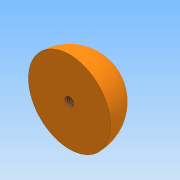
# Autodesk Inventor part: Ball_Upper Half
Saved by Autodesk Inventor 2018.1 (Build 221171000, 171)
## iProperties
Created: 2019-02-18
Part Number: Ball_Upper Half
Material: Nylon 6/6
Document SubType Name: Modeling
Designer: James
Density: 1.13 g/cm^3
Appearance: Orange
Author: James
Autodesk Inventor part; units mm, degrees
ref_plane "YZ Plane" through (0, 0, 0) normal (1, 0, 0) x (0, 1, 0)
ref_plane "XZ Plane" through (0, 0, 0) normal (0, 1, 0) x (-1, 0, 0)
ref_plane "XY Plane" through (0, 0, 0) normal (0, 0, 1) x (1, 0, 0)
sketch "Sketch1" plane through (0, 0, 0) normal (0, 0, 1) x (1, 0, 0)
  line L0 (0, 0) -> (0, 15)
  line L1 (0, 0) -> (15, 0)
  arc A0 (15, 0) -> (0, 15) centre (0, 0) ccw
  line L2 (0, -3.6213) -> (0, 21.7279) projected
  dimension "d2" = 15
  constraints: 4 end point, 2 coincident, 2 point on circle, 1 centre point, 1 horizontal, 1 vertical
  measures "d2" distance of L0.start L0.end
revolve "Revolution1" add sketch "Sketch1" angle 360 about axis through (0, -10, 0) along (0, 1, 0)
sketch "Sketch4" plane through (0, 0, 0) normal (0, -1, 0) x (1, 0, 0)
  point P0 (0, 0)
  point P1 (0, 0)
  constraints: 1 coincident
hole "Hole2" at (0, 0, 0) direction (0, 1, 0) diameter 3.242 depth 11.8 tip angle 118 thread size "M4x0.7" class "6H" standard "ANSI Metric M Profile"
shell "Shell2" [suppressed]
body "Solid1"
